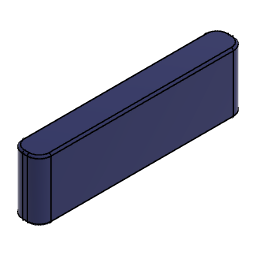
RB10PVC Battery (v1) (Autodesk Fusion 360 design; units mm, degrees)
Autodesk Fusion 360 part; units mm, degrees
sketch "Sketch1" plane through (0, 0, 0) normal (0, 0, 1) x (1, 0, 0)
  line L0 (0, 0) -> (36, 0)
  line L1 (36, 0) -> (36, 262)
  line L2 (36, 262) -> (0, 262)
  line L3 (0, 262) -> (0, 0)
  dimension "d1" = 36
  dimension "d2" = 262
  constraint horizontal L0
  constraint vertical L1
  constraint horizontal L2
  constraint vertical L3
  constraint coincident L0.start L3.end
  measures "d1" distance of L0.start L0.end
  measures "d2" distance of L0.start L2.end
extrude "Extrude1" add sketch "Sketch1" along normal blind 77
fillet "Fillet1" radius 15 4 edges at (36, 0, 38.5) (0, 0, 38.5) (36, 262, 38.5) (0, 262, 38.5)
fillet "Fillet2" radius 2.5 16 edges at (31.6066, 257.6066, 77) (18, 262, 77) (4.3934, 257.6066, 77) (0, 131, 77) (4.3934, 4.3934, 77) (18, 0, 77) (31.6066, 4.3934, 77) (36, 131, 77) (31.6066, 4.3934, 0) (36, 131, 0) (31.6066, 257.6066, 0) (18, 262, 0) (4.3934, 257.6066, 0) (0, 131, 0) (4.3934, 4.3934, 0) (18, 0, 0)
